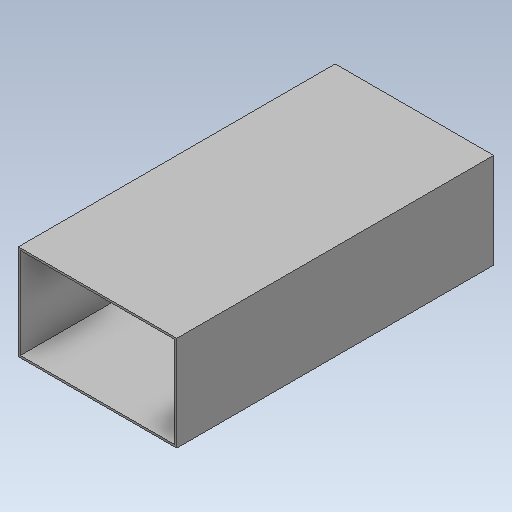
# Autodesk Inventor part: box
Saved by Autodesk Inventor 2021 (Build 250183000, 183)
## iProperties
RuleStatus: InUse
Created: 2017-08-03
Part Number: box
Material: Generic
Document SubType Name: Modeling
Designer: balglej
Density: 1 g/cm^3
Appearance: Carbon Fiber
length: 24.000 in
width: 40.000 in
height: 80.000 in
thickness: 0.500 in
Author: balglej
Autodesk Inventor part; units mm, degrees
ref_plane "YZ Plane" through (0, 0, 0) normal (1, 0, 0) x (0, 1, 0)
ref_plane "XZ Plane" through (0, 0, 0) normal (0, 1, 0) x (-1, 0, 0)
sketch "Sketch1" plane through (0, 0, 0) normal (0, 0, 1) x (1, 0, 0)
  line L0 (0, 0) -> (1016, 0)
  line L1 (1016, 0) -> (1016, 609.6)
  line L2 (1016, 609.6) -> (0, 609.6)
  line L3 (0, 609.6) -> (0, 0)
  line L4 (12.7, 12.7) -> (1003.3, 12.7)
  line L5 (1003.3, 12.7) -> (1003.3, 596.9)
  line L6 (1003.3, 596.9) -> (12.7, 596.9)
  line L7 (12.7, 596.9) -> (12.7, 12.7)
  dimension "d0" = 609.6
  dimension "d1" = 1016
  dimension "d2" = 12.7
  dimension "d3" = 12.7
  dimension "d4" = 12.7
  dimension "d5" = 12.7
  constraints: 16 end point, 4 parallel, 2 horizontal, 2 perpendicular
  measures "d0" distance of L0.end L1.end
  measures "d1" distance of L1.end L2.end
  measures "d2" distance between parallel lines of L3 L7
  measures "d3" distance between parallel lines of L2 L6
  measures "d4" distance between parallel lines of L0 L4
  measures "d5" distance between parallel lines of L1 L5
extrude "Extrusion1" add sketch "Sketch1" along normal blind 2032
extrude "Extrusion2" add sketch "Sketch1" along normal blind 12.7 contours L7 L6 L5 L4
ref_plane "Work Plane1" through (0, 304.8, 0) normal (0, -1, 0) x (1, 0, 0)
equation "\"d0\" = length"
equation "\"d1\" = width"
equation "\"d2\" = thickness"
equation "\"d3\" = thickness"
equation "\"d4\" = thickness"
equation "\"d5\" = thickness"
equation "\"d6\" = height"
equation "\"d8\" = thickness"
equation "\"length\" = 609.6"
equation "\"width\" = 1016"
equation "\"height\" = 2032"
equation "\"thickness\" = 12.7"
body "Solid1"
